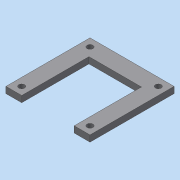
# Autodesk Inventor part: Camera-Holder_Mount-Bottom
Saved by Autodesk Inventor 2016 SP1 (Build 200210100, 210)
## iProperties
Created: 2016-02-08
Part Number: Camera-Holder_Mount-Bottom
Material: Generic
Document SubType Name: Modeling
Designer: Mohamed A.
Density: 1 g/cm^3
Appearance: Default
Author: Mohamed A.
Autodesk Inventor part; units mm, degrees
ref_plane "YZ Plane" through (0, 0, 0) normal (1, 0, 0) x (0, 1, 0)
ref_plane "XZ Plane" through (0, 0, 0) normal (0, 1, 0) x (-1, 0, 0)
ref_plane "XY Plane" through (0, 0, 0) normal (0, 0, 1) x (1, 0, 0)
sketch "Sketch1" plane through (0, 0, 0) normal (0, 0, 1) x (1, 0, 0)
  line L0 (-23.5, 23.5) -> (-23.5, -23.5) projected
  line L1 (23.5, 23.5) -> (-23.5, 23.5) projected
  line L2 (23.5, -23.5) -> (23.5, 23.5) projected
  line L3 (-23.5, -23.5) -> (23.5, -23.5) projected
  circle A0 centre (-18, -18) radius 1.4 projected
  circle A1 centre (-18, 18) radius 1.4 projected
  circle A2 centre (18, 18) radius 1.4 projected
  circle A3 centre (18, -18) radius 1.4 projected
  line L4 (12.5, 12) -> (12.5, -12) projected
  line L5 (-12.5, -12) -> (-12.5, 12) projected
  line L6 (-12.5, 12) -> (12.5, 12) projected
  line L7 (12.5, -12) -> (12.5, -23.5)
  line L8 (-12.5, -12) -> (-12.5, -23.5)
  point P0 (0, 0)
  constraints: 4 end point, 2 perpendicular, 2 point on line
extrude "Extrusion1" add sketch "Sketch1" along normal blind 3 contours L1 L2 L3 L7 L4 L6 L5 L8 L0
body "Solid1"
